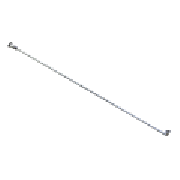
# Autodesk Inventor part: SpokeRear
Saved by Autodesk Inventor 2012 (Build 160160000, 160)
## iProperties
Created: 2001-05-08
Part Number: SpokeRear
Document SubType Name: Modeling
Designer: Administrator
Material: Default
Density: 1 g/cm^3
Control State: 0
Master: False
Checked Out: False
Shininess: 100.0
Length Units: 11272
Angle Units: 11279
Time Units: 11290
Mass Units: 11286
Length Display Precision: 3
Angle Display Precision: 2
Compacted: True
Density: 0.0
Volumn: 0.0
Area: 0.0
PropertySet Name: Model Information
Author: Administrator
Autodesk Inventor part; units mm, degrees
ref_plane "YZ Plane" through (0, 0, 0) normal (1, 0, 0) x (0, 1, 0)
ref_plane "XZ Plane" through (0, 0, 0) normal (0, 1, 0) x (-1, 0, 0)
ref_plane "XY Plane" through (0, 0, 0) normal (0, 0, 1) x (1, 0, 0)
sketch "Sketch1" plane through (0, 0, 0) normal (0, 0, 1) x (1, 0, 0)
  line L0 (-20.32, 1.016) -> (234.6305, 1.016)
  line L1 (-20.32, 1.016) -> (-20.32, 0)
  line L2 (-20.32, 0) -> (251.206, 0)
  line L3 (234.6305, 1.016) -> (235.8561, 1.524)
  line L4 (235.8561, 1.524) -> (251.206, 1.524)
  line L5 (251.206, 1.524) -> (251.206, 0)
  arc A0 (251.206, 1.524) -> (253.746, 4.064) centre (251.206, 4.064) ccw
  line L6 (253.746, 4.064) -> (253.746, 7.009)
  arc A1 (255.27, 7.9375) -> (251.9739, 7.75) centre (254.4821, -7.2764) ccw
  line L7 (253.746, 4.064) -> (256.794, 4.064)
  line L8 (255.27, 4.064) -> (255.27, 7.9375)
  arc A2 (251.206, 0) -> (255.27, 4.064) centre (251.206, 4.064) ccw
  line L9 (251.9739, 7.75) -> (251.9739, 7.3209)
  line L10 (251.9739, 7.3209) -> (253.746, 7.009)
  arc A3 (-19.626, 4.4916) -> (-20.32, 1.016) centre (-11.2701, 1.016) ccw
  line L11 (-19.626, 4.4916) -> (-19.3494, 4.4916)
  line L12 (-19.3494, 4.4916) -> (-18.8257, 3.175)
  line L13 (0, 3.175) -> (4.2213, 3.175)
  line L14 (4.2213, 3.175) -> (5.08, 1.016)
  line L15 (5.08, 1.016) -> (5.08, 0)
  line L16 (0, 3.175) -> (0, 0)
  line L17 (-18.8257, 3.175) -> (0, 3.175)
  line L18 (0, 0) -> (5.08, 0)
  dimension "d1" = 2.032
  dimension "d2" = 3.048
  dimension "d5" = 6.35
  dimension "d11" = 9.0499
  dimension "d12" = 25.4
  dimension "d13" = 5.08
  dimension "d14" = 0.2766
  dimension "d15" = 1.4943
  dimension "d16" = 1.2255
  dimension "d17" = 2.54
  dimension "d18" = 7.9375
  dimension "d19" = 15.2343
  dimension "d20" = 6.5922
  dimension "d21" = 275.59
  constraints: 38 end point, 8 parallel, 8 perpendicular, 8 point on circle, 4 centre point, 4 tangent, 3 point on line, 2 coincident, 1 horizontal, 1 midpoint
  measures "d1" diameter of L0 L2
  measures "d2" diameter of L4 L2
  measures "d5" diameter of L13 L2
  measures "d11" radius of A3
  measures "d12" distance between parallel lines of L15 L1
  measures "d13" distance between parallel lines of L15 L16
  measures "d14" distance of L11.start L11.end
  measures "d15" horizontal distance of L0.start L12.end
  measures "d16" horizontal distance of L0.end L3.end
  measures "d17" radius of A0
  measures "d18" distance from line of L8.end L2
  measures "d19" radius of A1
  measures "d20" diameter of L8 L9
  measures "d21" distance between parallel lines of L1 L8
revolve "Revolution1" add sketch "Sketch1" angle 360 about axis through (-20.32, 0, 0) along (1, 0, 0) contours L15 L2 L16 L0 | L0 L16 L13 L14 | L0 L3 L4 L5 L2 L15 | L16 L2 L1 L0 | L0 A3 L11 L12 L17 L16
sketch "Sketch3" plane through (0, 0, 0) normal (1, 0, 0) x (0, 1, 0)
  circle A0 centre (0, 0) radius 3.175 projected
  line L0 (2.2451, 2.2451) -> (-2.2451, 2.2451)
  line L1 (-2.2451, 2.2451) -> (-2.2451, -2.2451)
  line L2 (-2.2451, -2.2451) -> (2.2451, -2.2451)
  line L3 (2.2451, -2.2451) -> (2.2451, 2.2451)
  point P0 (-0.0045, 0)
  constraints: 8 end point, 4 point on circle, 2 parallel, 2 perpendicular, 1 horizontal
extrude "Extrusion1" cut sketch "Sketch3" along normal blind 7.9502 contours A0 L3 | L0 A0 | A0 L2 | L1 A0
revolve "Revolution2" add sketch "Sketch1" angle 360 about axis through (255.27, 4.064, 0) along (0, 1, 0) contours L7 L6 L10 L9 A1 L8
sketch "Sketch2" plane through (251.206, 0, 0) normal (1, 0, 0) x (0, 0, -1)
  circle A0 centre (0, 0) radius 1.524 projected
  line L0 (0, 4.064) -> (3.1623, 4.064)
  constraints: 2 end point, 1 horizontal
revolve "Revolution3" add sketch "Sketch2" angle 90 about axis through (251.206, 4.064, 0) along (0, 0, 1)
body "Solid1"
